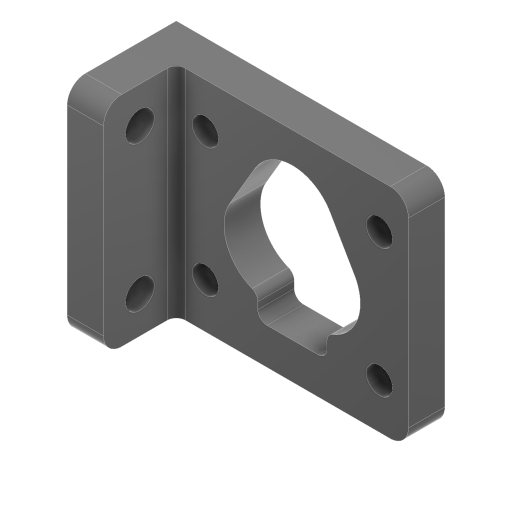
# Autodesk Inventor part: CAN Resistor Mount
Saved by Autodesk Inventor 2023 (Build 270158000, 158)
## iProperties
Created: 2023-12-17
Part Number: CAN Resistor Mount
Material: Generic
Document SubType Name: Modeling
Designer: Adam Arnold
Density: 1 g/cm^3
Appearance: Smooth - Black
Author: Adam Arnold
Autodesk Inventor part; units mm, degrees
ref_plane "YZ Plane" through (0, 0, 0) normal (1, 0, 0) x (0, 1, 0)
ref_plane "XZ Plane" through (0, 0, 0) normal (0, 1, 0) x (-1, 0, 0)
ref_plane "XY Plane" through (0, 0, 0) normal (0, 0, 1) x (1, 0, 0)
sketch "Sketch1" plane through (0, 0, 0) normal (0, 0, 1) x (1, 0, 0)
  line L0 (0, 0) -> (46.863, 0)
  line L1 (46.863, 0) -> (46.863, 38.1)
  line L2 (46.863, 38.1) -> (0, 38.1)
  line L3 (0, 38.1) -> (0, 0)
  dimension "d0" = 46.863
  dimension "d1" = 38.1
  constraints: 8 end point, 2 parallel, 1 horizontal, 1 perpendicular
  measures "d0" distance of L1.end L2.end
  measures "d1" distance of L0.end L1.end
extrude "Extrusion1" add sketch "Sketch1" along normal blind 6.35
sketch "Sketch2" plane through (0, 0, 6.35) normal (0, 0, 1) x (1, 0, 0)
  line L0 (46.863, 38.1) -> (0, 38.1) projected
  line L1 (0, 0) -> (46.863, 0) projected
  line L2 (0, 38.1) -> (6.35, 38.1)
  line L3 (6.35, 38.1) -> (6.35, 0)
  line L4 (6.35, 0) -> (0, 0)
  line L5 (0, 0) -> (0, 38.1)
  dimension "d4" = 6.35
  constraints: 8 end point, 2 parallel, 1 horizontal, 1 perpendicular, 1 point on line
  measures "d4" distance of L3.end L4.end
extrude "Extrusion2" add sketch "Sketch2" along normal blind 12.7
sketch "Sketch4" plane through (0, 0, 6.35) normal (0, 0, 1) x (1, 0, 0)
  line L0 (46.863, 38.1) -> (6.35, 38.1) projected
  line L1 (46.863, 0) -> (46.863, 38.1) projected
  point P0 (0, 0)
  point P1 (41.783, 30.2768)
  point P2 (40.513, 38.1)
  point P3 (6.35, 38.1)
  point P4 (43.688, 3.175)
  point P5 (43.688, 34.925)
  dimension "d8" = 7.8232
  dimension "d9" = 5.08
  constraints: 1 other
  measures "d8" distance from line of L0 point (41.783, 30.277)
hole "Hole1" at (41.783, 30.2768, 6.35) direction (0, 0, -1) diameter 4.572 end through all
sketch "Sketch5" plane through (0, 0, 6.35) normal (0, 0, 1) x (1, 0, 0)
  line L0 (6.35, 0) -> (46.863, 0) projected
  line L1 (46.863, 0) -> (46.863, 38.1) projected
  point P0 (0, 0)
  point P1 (41.783, 7.8232)
  point P2 (6.35, 0)
  point P3 (40.513, 0)
  point P4 (43.688, 3.175)
  point P5 (43.688, 34.925)
  dimension "d17" = 7.8232
  dimension "d18" = 5.08
  constraints: 1 other
  measures "d17" distance from line of L0 point (41.783, 7.823)
hole "Hole2" at (41.783, 7.8232, 6.35) direction (0, 0, -1) diameter 4.572 end through all
sketch "Sketch6" plane through (6.35, 0, 6.35) normal (1, 0, 0) x (0, 0, -1)
  line L0 (-12.7, 0) -> (-12.7, 38.1) projected
  line L1 (0, 38.1) -> (-12.7, 38.1) projected
  point P0 (6.35, 0)
  point P1 (-6.35, 31.75)
  dimension "d26" = 6.35
  dimension "d27" = 6.35
  measures "d26" distance from line of L0 point (-6.35, 31.75)
  measures "d27" distance from line of L1 point (-6.35, 31.75)
hole "Hole3" at (6.35, 31.75, 12.7) direction (-1, 0, 0) diameter 5.0038 end through all
sketch "Sketch7" plane through (6.35, 0, 6.35) normal (1, 0, 0) x (0, 0, -1)
  line L0 (-12.7, 0) -> (-12.7, 38.1) projected
  line L1 (0, 0) -> (-12.7, 0) projected
  point P0 (6.35, 0)
  point P1 (-6.35, 6.35)
  dimension "d35" = 6.35
  dimension "d36" = 6.35
  measures "d35" distance from line of L0 point (-6.35, 6.35)
  measures "d36" distance from line of L1 point (-6.35, 6.35)
hole "Hole4" at (6.35, 6.35, 12.7) direction (-1, 0, 0) diameter 5.0038 end through all
fillet "Fillet3" radius 3.175 4 edges at (3.175, 38.1, 19.05) (3.175, 0, 19.05) (46.863, 38.1, 3.175) (46.863, 0, 3.175)
fillet "Fillet4" radius 1.5875 1 edges at (6.35, 19.05, 6.35)
sketch "Sketch8" plane through (0, 0, 6.35) normal (0, 0, 1) x (1, 0, 0)
  line L0 (46.863, 3.175) -> (46.863, 34.925) projected
  line L1 (43.688, 38.1) -> (7.9375, 38.1) projected
  point P0 (0, 0)
  point P1 (11.4046, 30.2768)
  dimension "d47" = 35.4584
  dimension "d48" = 7.8232
  measures "d47" distance from line of L0 point (11.405, 30.277)
  measures "d48" distance from line of L1 point (11.405, 30.277)
hole "Hole5" at (11.4046, 30.2768, 6.35) direction (0, 0, -1) diameter 4.572 end through all
sketch "Sketch9" plane through (0, 0, 6.35) normal (0, 0, 1) x (1, 0, 0)
  line L0 (7.9375, 0) -> (43.688, 0) projected
  line L1 (46.863, 3.175) -> (46.863, 34.925) projected
  point P0 (0, 0)
  point P1 (11.4046, 7.8232)
  dimension "d56" = 7.8232
  dimension "d57" = 35.4584
  measures "d56" distance from line of L0 point (11.405, 7.823)
  measures "d57" distance from line of L1 point (11.405, 7.823)
hole "Hole6" at (11.4046, 7.8232, 6.35) direction (0, 0, -1) diameter 4.572 end through all
sketch "Sketch10" plane through (0, 0, 6.35) normal (0, 0, 1) x (1, 0, 0)
  line L0 (22.3774, 17.78) -> (30.8356, 17.78) construction
  line L1 (26.6065, 17.78) -> (26.6065, 25.1206) construction
  line L2 (46.863, 3.175) -> (46.863, 34.925) projected
  line L3 (7.9375, 0) -> (43.688, 0) projected
  line L4 (22.3774, 11.43) -> (30.8356, 11.43)
  line L5 (32.1087, 28.2905) -> (36.3378, 20.9499)
  arc A0 (32.8202, 23.8119) -> (26.6065, 13.0432) centre (30.8356, 17.78) ccw construction
  arc A1 (30.8356, 11.43) -> (36.3378, 20.9499) centre (30.8356, 17.78) ccw
  line L6 (21.1043, 28.2905) -> (16.8752, 20.9499)
  arc A2 (26.6065, 13.0432) -> (20.3928, 23.8119) centre (22.3774, 17.78) ccw construction
  arc A3 (16.8752, 20.9499) -> (22.3774, 11.43) centre (22.3774, 17.78) ccw
  arc A4 (32.1087, 28.2905) -> (21.1043, 28.2905) centre (26.6065, 25.1206) ccw
  arc A5 (20.3928, 23.8119) -> (32.8202, 23.8119) centre (26.6065, 25.1206) ccw construction
  line L7 (20.0039, 28.9245) -> (15.7157, 21.618)
  arc A6 (15.7157, 21.618) -> (20.574, 10.3063) centre (22.3774, 17.78) ccw
  arc A7 (32.639, 10.3765) -> (37.4382, 21.5839) centre (30.8356, 17.78) ccw
  line L8 (37.4382, 21.5839) -> (33.2091, 28.9245)
  arc A8 (33.2091, 28.9245) -> (20.0039, 28.9245) centre (26.6065, 25.1206) ccw
  line L9 (20.574, 6.35) -> (32.639, 6.35)
  line L10 (26.6065, 6.35) -> (26.6065, 4.7621) construction
  line L11 (20.574, 6.35) -> (20.574, 10.3063)
  line L12 (32.639, 6.35) -> (32.639, 10.3765)
  point P0 (0, 0)
  dimension "d65" = 8.4582
  dimension "d71" = 7.3406
  dimension "d72" = 20.2565
  dimension "d73" = 17.78
  dimension "d74" = 1.27
  dimension "d75" = 11.43
  dimension "d76" = 12.065
  dimension "d77" = 0
  constraints: 22 end point, 18 point on circle, 9 centre point, 6 tangent, 3 vertical, 2 horizontal, 2 midpoint, 1 coincident, 1 horizontal alignment, 1 parallel, 1 perpendicular, 1 other
  measures "d65" distance of L0.end L0.start
  measures "d71" distance of L1.start L1.end
  measures "d72" distance from line of L2 L1.start
  measures "d73" distance from line of L3 L1.start
  measures "d74" radial gap between concentric circles of A4 A8
  measures "d75" distance between parallel lines of L0 L9
  measures "d76" distance of L9.start L9.end
  measures "d77" distance from line of A4.centre L10
extrude "Extrusion3" cut sketch "Sketch10" against normal through all contours A3 L6 A4 L5 A1 L4 | A8 L8 A7 L12 L9 L11 A6 L7
fillet "Fillet5" radius 1.5875 2 edges at (20.574, 6.35, 3.175) (32.639, 6.35, 3.175)
fillet "Fillet6" radius 1.5875 2 edges at (20.574, 10.3063, 3.175) (32.639, 10.3765, 3.175)
body "Solid1"
